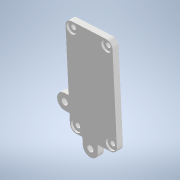
# Autodesk Inventor part: Пластина 2
Saved by Autodesk Inventor 2020 (Build 240168000, 168)
## iProperties
Created: 2020-12-07
Part Number: Пластина 2
Material: Типовые
Document SubType Name: Modeling
Designer: User
Density: 1 g/cm^3
Appearance: По умолчанию
Author: User
Autodesk Inventor part; units mm, degrees
ref_plane "YZ Plane" through (0, 0, 0) normal (1, 0, 0) x (0, 1, 0)
ref_plane "XZ Plane" through (0, 0, 0) normal (0, 1, 0) x (-1, 0, 0)
ref_plane "XY Plane" through (0, 0, 0) normal (0, 0, 1) x (1, 0, 0)
sketch "Эскиз1" plane through (0, 0, 0) normal (0, 0, 1) x (1, 0, 0)
  arc A0 (26.2085, -58.7088) -> (33.7788, -50.3011) centre (25.7898, -50.7198) ccw projected
  line L0 (26.2085, -58.7088) -> (8.1333, -59.6561) projected
  line L1 (28.0167, 59.648) -> (33.7788, -50.3011) projected
  arc A1 (28.0167, 59.648) -> (19.6089, 67.2184) centre (20.0276, 59.2293) ccw projected
  circle A2 centre (-2.0934, 39.9452) radius 12 projected
  circle A3 centre (0, 0) radius 12 projected
  line L2 (-29.998, -21.8425) -> (-34.0981, 56.3927) projected
  arc A4 (-35.8899, -22.1513) -> (-34.8432, -42.1239) centre (-35.3665, -32.1376) ccw projected
  line L3 (-29.998, -21.8425) -> (-35.8899, -22.1513) projected
  line L4 (-34.8432, -42.1239) -> (-28.9512, -41.8151) projected
  line L5 (-28.3359, -53.5564) -> (-28.9512, -41.8151) projected
  arc A5 (-28.3359, -53.5564) -> (-19.9282, -61.1267) centre (-20.3469, -53.1377) ccw projected
  line L6 (-11.8393, -60.7028) -> (-19.9282, -61.1267) projected
  arc A6 (-26.5277, 64.8005) -> (-34.0981, 56.3927) centre (-26.1091, 56.8114) ccw projected
  line L7 (-26.5277, 64.8005) -> (19.6089, 67.2184) projected
  arc A7 (-11.3817, -69.4335) -> (8.5909, -68.3868) centre (-1.3954, -68.9101) ccw projected
  line L8 (-11.8393, -60.7028) -> (-11.3817, -69.4335) projected
  line L9 (8.5909, -68.3868) -> (8.1333, -59.6561) projected
extrude "Выдавливание1" add sketch "Эскиз1" along normal blind 6
sketch "Эскиз2" plane through (0, 0, 6) normal (0, 0, 1) x (1, 0, 0)
  line L0 (33.7788, -50.3011) -> (28.0167, 59.648) projected
  line L1 (8.1333, -59.6561) -> (26.2085, -58.7088) projected
  arc A0 (26.2085, -58.7088) -> (33.7788, -50.3011) centre (25.7898, -50.7198) ccw projected
  arc A1 (-28.3359, -53.5564) -> (-19.9282, -61.1267) centre (-20.3469, -53.1377) ccw projected
  line L2 (-28.9512, -41.8151) -> (-28.3359, -53.5564) projected
  line L3 (-34.8432, -42.1239) -> (-28.9512, -41.8151) projected
  arc A2 (-35.8899, -22.1513) -> (-34.8432, -42.1239) centre (-35.3665, -32.1376) ccw projected
  line L4 (-34.0981, 56.3927) -> (-29.998, -21.8425) projected
  line L5 (-29.998, -21.8425) -> (-35.8899, -22.1513) projected
  arc A3 (-26.5277, 64.8005) -> (-34.0981, 56.3927) centre (-26.1091, 56.8114) ccw projected
  line L6 (19.6089, 67.2184) -> (-26.5277, 64.8005) projected
  arc A4 (28.0167, 59.648) -> (19.6089, 67.2184) centre (20.0276, 59.2293) ccw projected
  arc A5 (-11.3817, -69.4335) -> (8.5909, -68.3868) centre (-1.3954, -68.9101) ccw projected
  line L7 (-11.8393, -60.7028) -> (-11.3817, -69.4335) projected
  line L8 (-19.9282, -61.1267) -> (-11.8393, -60.7028) projected
  line L9 (8.5909, -68.3868) -> (8.1333, -59.6561) projected
  point P0 (0, 0)
extrude "Выдавливание2" add sketch "Эскиз2" along normal blind 2
sketch "Эскиз3" plane through (0, 0, 8) normal (0, 0, 1) x (1, 0, 0)
  circle A0 centre (20.0276, 59.2293) radius 3 construction
  circle A1 centre (-26.1091, 56.8114) radius 3 construction
  circle A2 centre (25.7898, -50.7198) radius 3 construction
  circle A3 centre (-20.3469, -53.1377) radius 3 construction
  point P0 (0, 0)
hole "Отверстие1" at (-20.3469, -53.1377, 8) at (25.7898, -50.7198, 8) at (-26.1091, 56.8114, 8) at (20.0276, 59.2293, 8) direction (0, 0, -1) diameter 6 end through all counterbore diameter 13.5 counterbore depth 2.5 clearance for "болты с шестигранной головкой / гайка ГОСТ 12876-67" size "M6" standard "ГОСТ"
sketch "Эскиз4" plane through (0, 0, 8) normal (0, 0, 1) x (1, 0, 0)
  circle A0 centre (-35.3665, -32.1376) radius 4 construction
  circle A1 centre (-1.3954, -68.9101) radius 4 construction
  point P0 (0, 0)
hole "Отверстие2" at (-35.3665, -32.1376, 8) at (-1.3954, -68.9101, 8) direction (0, 0, -1) diameter 8 end through all clearance for "с потайной головкой ГОСТ 12876-67" size "M8" standard "ГОСТ"
